Autodesk Fusion 360 part; units mm, degrees
note: some values were not read from the file. Set by a fixed rule: which sketch regions a step uses.
(part 7 of 14)
  spline S34 degree 5 poles (16.842, -9.555) (16.8421, -9.5551) (16.8422, -9.5551) (16.8424, -9.5553) (16.8428, -9.5555) (16.8433, -9.5558) (16.8439, -9.5561) (16.8446, -9.5565) (16.8454, -9.5569) (16.8462, -9.5573) (16.8472, -9.5578) (16.8482, -9.5584) (16.8493, -9.5589) (16.8504, -9.5596) (16.8517, -9.5602) (16.853, -9.5609) (16.8544, -9.5616) (16.8558, -9.5624) (16.8574, -9.5631) (16.859, -9.564) (16.8606, -9.5648) (16.8624, -9.5657) (16.8642, -9.5666) (16.8661, -9.5676) (16.8681, -9.5685) (16.8701, -9.5695) (16.8722, -9.5706) (16.8744, -9.5716) (16.8766, -9.5727) (16.8789, -9.5739) (16.8813, -9.575) (16.8837, -9.5762) (16.8863, -9.5774) (16.8888, -9.5786) (16.8915, -9.5798) (16.8942, -9.5811) (16.897, -9.5824) (16.8998, -9.5837) (16.9027, -9.5851) (16.9057, -9.5864) (16.9087, -9.5878) (16.9118, -9.5892) (16.9149, -9.5906) (16.9182, -9.5921) (16.9214, -9.5936) (16.9248, -9.5951) (16.9282, -9.5966) (16.9316, -9.5981) (16.9352, -9.5996) (16.9387, -9.6012) (16.9424, -9.6028) (16.9461, -9.6044) (16.9499, -9.606) (16.9537, -9.6076) (16.9576, -9.6093) (16.9615, -9.6109) (16.9655, -9.6126) (16.9695, -9.6143) (16.9737, -9.616) (16.9778, -9.6177) (16.982, -9.6195) (16.9863, -9.6212) (16.9907, -9.623) (16.9951, -9.6248) (16.9995, -9.6266) (17.004, -9.6284) (17.0086, -9.6302) (17.0132, -9.632) (17.0178, -9.6339) (17.0226, -9.6357) (17.0273, -9.6376) (17.0322, -9.6395) (17.0371, -9.6413) (17.042, -9.6432) (17.047, -9.6451) (17.052, -9.6471) (17.0571, -9.649) (17.0623, -9.6509) (17.0675, -9.6528) (17.0727, -9.6548) (17.078, -9.6568) (17.0834, -9.6587) (17.0888, -9.6607) (17.0942, -9.6627) (17.0997, -9.6647) (17.1053, -9.6667) (17.1109, -9.6687) (17.1166, -9.6707) (17.1223, -9.6727) (17.128, -9.6747) (17.1338, -9.6767) (17.1397, -9.6788) (17.1456, -9.6808) (17.1515, -9.6828) (17.1575, -9.6849) (17.1636, -9.6869) (17.1697, -9.689) (17.1758, -9.6911) (17.182, -9.6931) (17.1882, -9.6952) (17.1945, -9.6973) (17.2009, -9.6993) (17.2072, -9.7014) (17.2137, -9.7035) (17.2201, -9.7056) (17.2267, -9.7077) (17.2332, -9.7098) (17.2398, -9.7119) (17.2465, -9.714) (17.2532, -9.7161) (17.2599, -9.7181) (17.2667, -9.7202) (17.2736, -9.7223) (17.2805, -9.7244) (17.2874, -9.7265) (17.2944, -9.7287) (17.3014, -9.7308) (17.3084, -9.7329) (17.3155, -9.735) (17.3227, -9.7371) (17.3299, -9.7392) (17.3371, -9.7413) (17.3444, -9.7434) (17.3517, -9.7455) (17.3591, -9.7476) (17.3665, -9.7497) (17.3739, -9.7518) (17.3814, -9.7539) (17.389, -9.756) (17.3966, -9.7581) (17.4042, -9.7602) (17.4118, -9.7622) (17.4195, -9.7643) (17.4273, -9.7664) (17.4351, -9.7685) (17.4429, -9.7706) (17.4508, -9.7727) (17.4587, -9.7747) (17.4666, -9.7768) (17.4746, -9.7789) (17.4827, -9.7809) (17.4907, -9.783) (17.4988, -9.785) (17.507, -9.7871) (17.5152, -9.7892) (17.5234, -9.7912) (17.5317, -9.7932) (17.54, -9.7953) (17.5484, -9.7973) (17.5568, -9.7993) (17.5652, -9.8014) (17.5737, -9.8034) (17.5822, -9.8054) (17.5907, -9.8074) (17.5993, -9.8094) (17.6079, -9.8114) (17.6166, -9.8134) (17.6253, -9.8154) (17.634, -9.8174) (17.6428, -9.8193) (17.6516, -9.8213) (17.6605, -9.8233) (17.6694, -9.8252) (17.6783, -9.8272) (17.6873, -9.8291) (17.6963, -9.831) (17.7053, -9.833) (17.7144, -9.8349) (17.7235, -9.8368) (17.7326, -9.8387) (17.7418, -9.8406) (17.751, -9.8425) (17.7603, -9.8444) (17.7696, -9.8463) (17.7789, -9.8481) (17.7883, -9.85) (17.7977, -9.8519) (17.8071, -9.8537) (17.8166, -9.8555) (17.8261, -9.8574) (17.8357, -9.8592) (17.8453, -9.861) (17.8549, -9.8628) (17.8645, -9.8646) (17.8742, -9.8664) (17.8839, -9.8682) (17.8937, -9.8699) (17.9035, -9.8717) (17.9133, -9.8735) (17.9232, -9.8752) (17.9331, -9.8769) (17.943, -9.8787) (17.9529, -9.8804) (17.9629, -9.8821) (17.973, -9.8838) (17.983, -9.8855) (17.9931, -9.8871) (18.0033, -9.8888) (18.0134, -9.8904) (18.0236, -9.8921) (18.0339, -9.8937) (18.0441, -9.8953) (18.0544, -9.897) (18.0647, -9.8986) (18.0751, -9.9002) (18.0855, -9.9017) (18.0959, -9.9033) (18.1064, -9.9049) (18.1169, -9.9064) (18.1274, -9.9079) (18.138, -9.9095) (18.1486, -9.911) (18.1592, -9.9125) (18.1698, -9.914) (18.1805, -9.9155) (18.1912, -9.9169) (18.202, -9.9184) (18.2128, -9.9198) (18.2236, -9.9213) (18.2344, -9.9227) (18.2453, -9.9241) (18.2562, -9.9255) (18.2671, -9.9269) (18.2781, -9.9282) (18.2891, -9.9296) (18.3001, -9.9309) (18.3112, -9.9323) (18.3223, -9.9336) (18.3334, -9.9349) (18.3445, -9.9362) (18.3557, -9.9375) (18.3669, -9.9387) (18.3782, -9.94) (18.3894, -9.9412) (18.4007, -9.9425) (18.4121, -9.9437) (18.4234, -9.9449) (18.4348, -9.9461) (18.4462, -9.9473) (18.4577, -9.9484) (18.4691, -9.9496) (18.4783, -9.9505) (18.4853, -9.9512) (18.4899, -9.9516) (18.4922, -9.9518) knots 0 0 0 0 0 0 0.00416667 0.00833333 0.0125 0.01666667 0.02083333 0.025 0.02916667 0.03333333 0.0375 0.04166667 0.04583333 0.05 0.05416667 0.05833333 0.0625 0.06666667 0.07083333 0.075 0.07916667 0.08333333 0.0875 0.09166667 0.09583333 0.1 0.10416667 0.10833333 0.1125 0.11666667 0.12083333 0.125 0.12916667 0.13333333 0.1375 0.14166667 0.14583333 0.15 0.15416667 0.15833333 0.1625 0.16666667 0.17083333 0.175 0.17916667 0.18333333 0.1875 0.19166667 0.19583333 0.2 0.20416667 0.20833333 0.2125 0.21666667 0.22083333 0.225 0.22916667 0.23333333 0.2375 0.24166667 0.24583333 0.25 0.25416667 0.25833333 0.2625 0.26666667 0.27083333 0.275 0.27916667 0.28333333 0.2875 0.29166667 0.29583333 0.3 0.30416667 0.30833333 0.3125 0.31666667 0.32083333 0.325 0.32916667 0.33333333 0.3375 0.34166667 0.34583333 0.35 0.35416667 0.35833333 0.3625 0.36666667 0.37083333 0.375 0.37916667 0.38333333 0.3875 0.39166667 0.39583333 0.4 0.40416667 0.40833333 0.4125 0.41666667 0.42083333 0.425 0.42916667 0.43333333 0.4375 0.44166667 0.44583333 0.45 0.45416667 0.45833333 0.4625 0.46666667 0.47083333 0.475 0.47916667 0.48333333 0.4875 0.49166667 0.49583333 0.5 0.50416667 0.50833333 0.5125 0.51666667 0.52083333 0.525 0.52916667 0.53333333 0.5375 0.54166667 0.54583333 0.55 0.55416667 0.55833333 0.5625 0.56666667 0.57083333 0.575 0.57916667 0.58333333 0.5875 0.59166667 0.59583333 0.6 0.60416667 0.60833333 0.6125 0.61666667 0.62083333 0.625 0.62916667 0.63333333 0.6375 0.64166667 0.64583333 0.65 0.65416667 0.65833333 0.6625 0.66666667 0.67083333 0.675 0.67916667 0.68333333 0.6875 0.69166667 0.69583333 0.7 0.70416667 0.70833333 0.7125 0.71666667 0.72083333 0.725 0.72916667 0.73333333 0.7375 0.74166667 0.74583333 0.75 0.75416667 0.75833333 0.7625 0.76666667 0.77083333 0.775 0.77916667 0.78333333 0.7875 0.79166667 0.79583333 0.8 0.80416667 0.80833333 0.8125 0.81666667 0.82083333 0.825 0.82916667 0.83333333 0.8375 0.84166667 0.84583333 0.85 0.85416667 0.85833333 0.8625 0.86666667 0.87083333 0.875 0.87916667 0.88333333 0.8875 0.89166667 0.89583333 0.9 0.90416667 0.90833333 0.9125 0.91666667 0.92083333 0.925 0.92916667 0.93333333 0.9375 0.94166667 0.94583333 0.95 0.95416667 0.95833333 0.9625 0.96666667 0.97083333 0.975 0.97916667 0.98333333 0.9875 0.99166667 0.99583333 1 1 1 1 1 1
  arc A35 (18.4922, -9.9518) -> (18.9206, -9.111) centre (0, 0) ccw
  spline S35 degree 5 poles (18.9206, -9.111) (18.9191, -9.1092) (18.916, -9.1058) (18.9114, -9.1006) (18.9053, -9.0936) (18.8976, -9.085) (18.8899, -9.0765) (18.8823, -9.0679) (18.8746, -9.0594) (18.8669, -9.0509) (18.8593, -9.0425) (18.8517, -9.034) (18.844, -9.0257) (18.8364, -9.0173) (18.8288, -9.009) (18.8212, -9.0007) (18.8136, -8.9924) (18.806, -8.9842) (18.7984, -8.976) (18.7908, -8.9678) (18.7833, -8.9597) (18.7757, -8.9516) (18.7681, -8.9436) (18.7606, -8.9355) (18.7531, -8.9275) (18.7455, -8.9195) (18.738, -8.9116) (18.7305, -8.9037) (18.723, -8.8958) (18.7155, -8.888) (18.708, -8.8802) (18.7005, -8.8724) (18.6931, -8.8647) (18.6856, -8.857) (18.6782, -8.8493) (18.6707, -8.8416) (18.6633, -8.834) (18.6559, -8.8264) (18.6485, -8.8189) (18.6411, -8.8114) (18.6337, -8.8039) (18.6263, -8.7965) (18.6189, -8.789) (18.6116, -8.7817) (18.6042, -8.7743) (18.5969, -8.767) (18.5896, -8.7597) (18.5823, -8.7525) (18.575, -8.7452) (18.5677, -8.7381) (18.5604, -8.7309) (18.5531, -8.7238) (18.5459, -8.7167) (18.5386, -8.7096) (18.5314, -8.7026) (18.5242, -8.6956) (18.517, -8.6887) (18.5098, -8.6818) (18.5026, -8.6749) (18.4954, -8.668) (18.4883, -8.6612) (18.4811, -8.6544) (18.474, -8.6477) (18.4669, -8.641) (18.4598, -8.6343) (18.4527, -8.6276) (18.4456, -8.621) (18.4386, -8.6144) (18.4315, -8.6079) (18.4245, -8.6013) (18.4175, -8.5949) (18.4105, -8.5884) (18.4035, -8.582) (18.3966, -8.5756) (18.3896, -8.5693) (18.3827, -8.5629) (18.3757, -8.5567) (18.3688, -8.5504) (18.3619, -8.5442) (18.3551, -8.538) (18.3482, -8.5319) (18.3414, -8.5258) (18.3346, -8.5197) (18.3277, -8.5137) (18.321, -8.5076) (18.3142, -8.5017) (18.3074, -8.4957) (18.3007, -8.4898) (18.294, -8.4839) (18.2873, -8.4781) (18.2806, -8.4723) (18.2739, -8.4665) (18.2673, -8.4608) (18.2606, -8.4551) (18.254, -8.4494) (18.2474, -8.4438) (18.2409, -8.4382) (18.2343, -8.4326) (18.2278, -8.4271) (18.2213, -8.4216) (18.2148, -8.4162) (18.2083, -8.4107) (18.2018, -8.4054) (18.1954, -8.4) (18.189, -8.3947) (18.1826, -8.3894) (18.1762, -8.3841) (18.1699, -8.3789) (18.1635, -8.3737) (18.1572, -8.3686) (18.151, -8.3635) (18.1447, -8.3584) (18.1385, -8.3534) (18.1322, -8.3484) (18.126, -8.3434) (18.1199, -8.3385) (18.1137, -8.3336) (18.1076, -8.3287) (18.1015, -8.3239) (18.0954, -8.3191) (18.0894, -8.3143) (18.0833, -8.3096) (18.0773, -8.3049) (18.0714, -8.3003) (18.0654, -8.2956) (18.0595, -8.291) (18.0536, -8.2865) (18.0477, -8.282) (18.0418, -8.2775) (18.036, -8.2731) (18.0302, -8.2687) (18.0244, -8.2643) (18.0187, -8.26) (18.013, -8.2557) (18.0073, -8.2514) (18.0016, -8.2472) (17.996, -8.243) (17.9904, -8.2388) (17.9848, -8.2347) (17.9793, -8.2306) (17.9737, -8.2266) (17.9682, -8.2226) (17.9628, -8.2186) (17.9573, -8.2147) (17.9519, -8.2108) (17.9466, -8.2069) (17.9412, -8.2031) (17.9359, -8.1993) (17.9306, -8.1955) (17.9254, -8.1918) (17.9202, -8.1881) (17.915, -8.1844) (17.9098, -8.1808) (17.9047, -8.1772) (17.8996, -8.1737) (17.8946, -8.1702) (17.8896, -8.1667) (17.8846, -8.1633) (17.8796, -8.1599) (17.8747, -8.1565) (17.8698, -8.1532) (17.865, -8.1499) (17.8602, -8.1467) (17.8554, -8.1435) (17.8507, -8.1403) (17.846, -8.1372) (17.8413, -8.1341) (17.8367, -8.131) (17.8321, -8.128) (17.8276, -8.125) (17.823, -8.122) (17.8186, -8.1191) (17.8141, -8.1162) (17.8097, -8.1134) (17.8054, -8.1106) (17.8011, -8.1078) (17.7968, -8.1051) (17.7926, -8.1024) (17.7884, -8.0997) (17.7842, -8.0971) (17.7801, -8.0945) (17.7761, -8.092) (17.772, -8.0895) (17.7681, -8.087) (17.7641, -8.0846) (17.7602, -8.0822) (17.7564, -8.0798) (17.7526, -8.0775) (17.7488, -8.0752) (17.7451, -8.073) (17.7415, -8.0708) (17.7378, -8.0686) (17.7343, -8.0665) (17.7308, -8.0644) (17.7273, -8.0623) (17.7239, -8.0603) (17.7205, -8.0583) (17.7172, -8.0564) (17.7139, -8.0545) (17.7107, -8.0526) (17.7075, -8.0508) (17.7044, -8.049) (17.7013, -8.0472) (17.6983, -8.0455) (17.6954, -8.0438) (17.6925, -8.0422) (17.6896, -8.0406) (17.6868, -8.0391) (17.6841, -8.0375) (17.6814, -8.0361) (17.6788, -8.0346) (17.6762, -8.0332) (17.6737, -8.0318) (17.6713, -8.0305) (17.6689, -8.0292) (17.6666, -8.028) (17.6643, -8.0268) (17.6621, -8.0256) (17.66, -8.0245) (17.6579, -8.0234) (17.6559, -8.0223) (17.654, -8.0213) (17.6521, -8.0203) (17.6503, -8.0194) (17.6485, -8.0185) (17.6469, -8.0176) (17.6452, -8.0168) (17.6437, -8.016) (17.6422, -8.0153) (17.6408, -8.0146) (17.6395, -8.0139) (17.6383, -8.0133) (17.6371, -8.0127) (17.636, -8.0122) (17.635, -8.0117) (17.634, -8.0112) (17.6332, -8.0108) (17.6324, -8.0104) (17.6317, -8.0101) (17.631, -8.0098) (17.6305, -8.0095) (17.6301, -8.0094) (17.6299, -8.0093) (17.6297, -8.0092) (17.6297, -8.0092) knots -1 -1 -1 -1 -1 -1 -0.99583333 -0.99166667 -0.9875 -0.98333333 -0.97916667 -0.975 -0.97083333 -0.96666667 -0.9625 -0.95833333 -0.95416667 -0.95 -0.94583333 -0.94166667 -0.9375 -0.93333333 -0.92916667 -0.925 -0.92083333 -0.91666667 -0.9125 -0.90833333 -0.90416667 -0.9 -0.89583333 -0.89166667 -0.8875 -0.88333333 -0.87916667 -0.875 -0.87083333 -0.86666667 -0.8625 -0.85833333 -0.85416667 -0.85 -0.84583333 -0.84166667 -0.8375 -0.83333333 -0.82916667 -0.825 -0.82083333 -0.81666667 -0.8125 -0.80833333 -0.80416667 -0.8 -0.79583333 -0.79166667 -0.7875 -0.78333333 -0.77916667 -0.775 -0.77083333 -0.76666667 -0.7625 -0.75833333 -0.75416667 -0.75 -0.74583333 -0.74166667 -0.7375 -0.73333333 -0.72916667 -0.725 -0.72083333 -0.71666667 -0.7125 -0.70833333 -0.70416667 -0.7 -0.69583333 -0.69166667 -0.6875 -0.68333333 -0.67916667 -0.675 -0.67083333 -0.66666667 -0.6625 -0.65833333 -0.65416667 -0.65 -0.64583333 -0.64166667 -0.6375 -0.63333333 -0.62916667 -0.625 -0.62083333 -0.61666667 -0.6125 -0.60833333 -0.60416667 -0.6 -0.59583333 -0.59166667 -0.5875 -0.58333333 -0.57916667 -0.575 -0.57083333 -0.56666667 -0.5625 -0.55833333 -0.55416667 -0.55 -0.54583333 -0.54166667 -0.5375 -0.53333333 -0.52916667 -0.525 -0.52083333 -0.51666667 -0.5125 -0.50833333 -0.50416667 -0.5 -0.49583333 -0.49166667 -0.4875 -0.48333333 -0.47916667 -0.475 -0.47083333 -0.46666667 -0.4625 -0.45833333 -0.45416667 -0.45 -0.44583333 -0.44166667 -0.4375 -0.43333333 -0.42916667 -0.425 -0.42083333 -0.41666667 -0.4125 -0.40833333 -0.40416667 -0.4 -0.39583333 -0.39166667 -0.3875 -0.38333333 -0.37916667 -0.375 -0.37083333 -0.36666667 -0.3625 -0.35833333 -0.35416667 -0.35 -0.34583333 -0.34166667 -0.3375 -0.33333333 -0.32916667 -0.325 -0.32083333 -0.31666667 -0.3125 -0.30833333 -0.30416667 -0.3 -0.29583333 -0.29166667 -0.2875 -0.28333333 -0.27916667 -0.275 -0.27083333 -0.26666667 -0.2625 -0.25833333 -0.25416667 -0.25 -0.24583333 -0.24166667 -0.2375 -0.23333333 -0.22916667 -0.225 -0.22083333 -0.21666667 -0.2125 -0.20833333 -0.20416667 -0.2 -0.19583333 -0.19166667 -0.1875 -0.18333333 -0.17916667 -0.175 -0.17083333 -0.16666667 -0.1625 -0.15833333 -0.15416667 -0.15 -0.14583333 -0.14166667 -0.1375 -0.13333333 -0.12916667 -0.125 -0.12083333 -0.11666667 -0.1125 -0.10833333 -0.10416667 -0.1 -0.09583333 -0.09166667 -0.0875 -0.08333333 -0.07916667 -0.075 -0.07083333 -0.06666667 -0.0625 -0.05833333 -0.05416667 -0.05 -0.04583333 -0.04166667 -0.0375 -0.03333333 -0.02916667 -0.025 -0.02083333 -0.01666667 -0.0125 -0.00833333 -0.00416667 0 0 0 0 0 0
  line L70 (17.6297, -8.0092) -> (17.629, -8.0089)
  line L71 (17.629, -8.0089) -> (17.0709, -7.7553)
  arc A36 (17.0709, -7.7553) -> (17.5548, -6.5871) centre (0, 0) ccw
  line L72 (17.5548, -6.5871) -> (18.1287, -6.8025)
  line L73 (18.1287, -6.8025) -> (18.1294, -6.8027)
  spline S36 degree 5 poles (18.1294, -6.8027) (18.1295, -6.8027) (18.1296, -6.8028) (18.1298, -6.8029) (18.1302, -6.803) (18.1308, -6.8032) (18.1315, -6.8035) (18.1322, -6.8037) (18.133, -6.804) (18.1339, -6.8043) (18.1349, -6.8047) (18.136, -6.8051) (18.1372, -6.8055) (18.1384, -6.8059) (18.1397, -6.8063) (18.1411, -6.8068) (18.1426, -6.8073) (18.1442, -6.8078) (18.1458, -6.8083) (18.1475, -6.8089) (18.1493, -6.8095) (18.1512, -6.8101) (18.1531, -6.8107) (18.1552, -6.8113) (18.1572, -6.812) (18.1594, -6.8127) (18.1617, -6.8134) (18.164, -6.8141) (18.1663, -6.8148) (18.1688, -6.8155) (18.1713, -6.8163) (18.1739, -6.8171) (18.1766, -6.8179) (18.1793, -6.8187) (18.1821, -6.8195) (18.185, -6.8203) (18.1879, -6.8212) (18.191, -6.822) (18.194, -6.8229) (18.1972, -6.8238) (18.2004, -6.8247) (18.2037, -6.8256) (18.207, -6.8265) (18.2104, -6.8274) (18.2139, -6.8284) (18.2174, -6.8293) (18.221, -6.8303) (18.2247, -6.8312) (18.2284, -6.8322) (18.2322, -6.8332) (18.236, -6.8342) (18.2399, -6.8352) (18.2439, -6.8362) (18.2479, -6.8372) (18.252, -6.8382) (18.2561, -6.8392) (18.2604, -6.8403) (18.2646, -6.8413) (18.269, -6.8424) (18.2733, -6.8434) (18.2778, -6.8445) (18.2823, -6.8455) (18.2868, -6.8466) (18.2915, -6.8477) (18.2961, -6.8487) (18.3009, -6.8498) (18.3057, -6.8509) (18.3105, -6.852) (18.3154, -6.8531) (18.3203, -6.8542) (18.3254, -6.8553) (18.3304, -6.8564) (18.3355, -6.8575) (18.3407, -6.8586) (18.3459, -6.8597) (18.3512, -6.8608) (18.3565, -6.8619) (18.3619, -6.863) (18.3674, -6.8641) (18.3729, -6.8652) (18.3784, -6.8663) (18.384, -6.8674) (18.3896, -6.8685) (18.3953, -6.8696) (18.4011, -6.8707) (18.4069, -6.8718) (18.4127, -6.8729) (18.4186, -6.874) (18.4246, -6.8751) (18.4306, -6.8762) (18.4366, -6.8773) (18.4427, -6.8784) (18.4489, -6.8795) (18.4551, -6.8805) (18.4613, -6.8816) (18.4676, -6.8827) (18.474, -6.8838) (18.4804, -6.8849) (18.4868, -6.8859) (18.4933, -6.887) (18.4998, -6.8881) (18.5064, -6.8891) (18.513, -6.8902) (18.5197, -6.8912) (18.5264, -6.8923) (18.5332, -6.8933) (18.54, -6.8944) (18.5469, -6.8954) (18.5538, -6.8964) (18.5607, -6.8974) (18.5677, -6.8985) (18.5747, -6.8995) (18.5818, -6.9005) (18.5889, -6.9015) (18.5961, -6.9025) (18.6033, -6.9034) (18.6106, -6.9044) (18.6179, -6.9054) (18.6252, -6.9064) (18.6326, -6.9073) (18.6401, -6.9083) (18.6475, -6.9092) (18.6551, -6.9102) (18.6626, -6.9111) (18.6702, -6.912) (18.6779, -6.9129) (18.6856, -6.9138) (18.6933, -6.9147) (18.7011, -6.9156) (18.7089, -6.9165) (18.7167, -6.9174) (18.7246, -6.9182) (18.7326, -6.9191) (18.7405, -6.9199) (18.7485, -6.9208) (18.7566, -6.9216) (18.7647, -6.9224) (18.7728, -6.9232) (18.781, -6.924) (18.7892, -6.9248) (18.7975, -6.9256) (18.8058, -6.9264) (18.8141, -6.9272) (18.8225, -6.9279) (18.8309, -6.9287) (18.8394, -6.9294) (18.8479, -6.9301) (18.8564, -6.9308) (18.8649, -6.9315) (18.8736, -6.9322) (18.8822, -6.9329) (18.8909, -6.9336) (18.8996, -6.9342) (18.9084, -6.9349) (18.9171, -6.9355) (18.926, -6.9361) (18.9348, -6.9367) (18.9438, -6.9373) (18.9527, -6.9379) (18.9617, -6.9385) (18.9707, -6.9391) (18.9797, -6.9396) (18.9888, -6.9402) (18.9979, -6.9407) (19.0071, -6.9412) (19.0163, -6.9417) (19.0255, -6.9422) (19.0348, -6.9427) (19.0441, -6.9431) (19.0534, -6.9436) (19.0628, -6.944) (19.0722, -6.9445) (19.0816, -6.9449) (19.0911, -6.9453) (19.1006, -6.9457) (19.1102, -6.946) (19.1198, -6.9464) (19.1294, -6.9467) (19.139, -6.9471) (19.1487, -6.9474) (19.1584, -6.9477) (19.1681, -6.948) (19.1779, -6.9483) (19.1877, -6.9485) (19.1976, -6.9488) (19.2075, -6.949) (19.2174, -6.9492) (19.2273, -6.9495) (19.2373, -6.9496) (19.2473, -6.9498) (19.2574, -6.95) (19.2674, -6.9501) (19.2775, -6.9503) (19.2877, -6.9504) (19.2979, -6.9505) (19.3081, -6.9506) (19.3183, -6.9507) (19.3286, -6.9507) (19.3389, -6.9508) (19.3492, -6.9508) (19.3595, -6.9508) (19.3699, -6.9508) (19.3804, -6.9508) (19.3908, -6.9507) (19.4013, -6.9507) (19.4118, -6.9506) (19.4224, -6.9505) (19.4329, -6.9505) (19.4435, -6.9503) (19.4542, -6.9502) (19.4648, -6.9501) (19.4755, -6.9499) (19.4863, -6.9497) (19.497, -6.9495) (19.5078, -6.9493) (19.5186, -6.9491) (19.5295, -6.9488) (19.5403, -6.9486) (19.5512, -6.9483) (19.5622, -6.948) (19.5731, -6.9477) (19.5841, -6.9474) (19.5951, -6.947) (19.6062, -6.9467) (19.6172, -6.9463) (19.6283, -6.9459) (19.6395, -6.9455) (19.6506, -6.9451) (19.6618, -6.9446) (19.673, -6.9441) (19.6843, -6.9437) (19.6956, -6.9432) (19.7068, -6.9426) (19.7182, -6.9421) (19.7295, -6.9416) (19.7409, -6.941) (19.7523, -6.9404) (19.7637, -6.9398) (19.7752, -6.9392) (19.7867, -6.9385) (19.7982, -6.9379) (19.8074, -6.9373) (19.8144, -6.9369) (19.819, -6.9366) (19.8213, -6.9365) knots 0 0 0 0 0 0 0.00416667 0.00833333 0.0125 0.01666667 0.02083333 0.025 0.02916667 0.03333333 0.0375 0.04166667 0.04583333 0.05 0.05416667 0.05833333 0.0625 0.06666667 0.07083333 0.075 0.07916667 0.08333333 0.0875 0.09166667 0.09583333 0.1 0.10416667 0.10833333 0.1125 0.11666667 0.12083333 0.125 0.12916667 0.13333333 0.1375 0.14166667 0.14583333 0.15 0.15416667 0.15833333 0.1625 0.16666667 0.17083333 0.175 0.17916667 0.18333333 0.1875 0.19166667 0.19583333 0.2 0.20416667 0.20833333 0.2125 0.21666667 0.22083333 0.225 0.22916667 0.23333333 0.2375 0.24166667 0.24583333 0.25 0.25416667 0.25833333 0.2625 0.26666667 0.27083333 0.275 0.27916667 0.28333333 0.2875 0.29166667 0.29583333 0.3 0.30416667 0.30833333 0.3125 0.31666667 0.32083333 0.325 0.32916667 0.33333333 0.3375 0.34166667 0.34583333 0.35 0.35416667 0.35833333 0.3625 0.36666667 0.37083333 0.375 0.37916667 0.38333333 0.3875 0.39166667 0.39583333 0.4 0.40416667 0.40833333 0.4125 0.41666667 0.42083333 0.425 0.42916667 0.43333333 0.4375 0.44166667 0.44583333 0.45 0.45416667 0.45833333 0.4625 0.46666667 0.47083333 0.475 0.47916667 0.48333333 0.4875 0.49166667 0.49583333 0.5 0.50416667 0.50833333 0.5125 0.51666667 0.52083333 0.525 0.52916667 0.53333333 0.5375 0.54166667 0.54583333 0.55 0.55416667 0.55833333 0.5625 0.56666667 0.57083333 0.575 0.57916667 0.58333333 0.5875 0.59166667 0.59583333 0.6 0.60416667 0.60833333 0.6125 0.61666667 0.62083333 0.625 0.62916667 0.63333333 0.6375 0.64166667 0.64583333 0.65 0.65416667 0.65833333 0.6625 0.66666667 0.67083333 0.675 0.67916667 0.68333333 0.6875 0.69166667 0.69583333 0.7 0.70416667 0.70833333 0.7125 0.71666667 0.72083333 0.725 0.72916667 0.73333333 0.7375 0.74166667 0.74583333 0.75 0.75416667 0.75833333 0.7625 0.76666667 0.77083333 0.775 0.77916667 0.78333333 0.7875 0.79166667 0.79583333 0.8 0.80416667 0.80833333 0.8125 0.81666667 0.82083333 0.825 0.82916667 0.83333333 0.8375 0.84166667 0.84583333 0.85 0.85416667 0.85833333 0.8625 0.86666667 0.87083333 0.875 0.87916667 0.88333333 0.8875 0.89166667 0.89583333 0.9 0.90416667 0.90833333 0.9125 0.91666667 0.92083333 0.925 0.92916667 0.93333333 0.9375 0.94166667 0.94583333 0.95 0.95416667 0.95833333 0.9625 0.96666667 0.97083333 0.975 0.97916667 0.98333333 0.9875 0.99166667 0.99583333 1 1 1 1 1 1
  arc A37 (19.8213, -6.9365) -> (20.113, -6.039) centre (0, 0) ccw
  spline S37 degree 5 poles (20.113, -6.039) (20.1112, -6.0375) (20.1076, -6.0345) (20.1022, -6.0301) (20.0951, -6.0242) (20.0861, -6.0169) (20.0772, -6.0097) (20.0683, -6.0024) (20.0594, -5.9952) (20.0505, -5.988) (20.0417, -5.9809) (20.0328, -5.9738) (20.024, -5.9667) (20.0151, -5.9596) (20.0063, -5.9526) (19.9975, -5.9456) (19.9887, -5.9386) (19.9799, -5.9317) (19.9711, -5.9248) (19.9624, -5.9179) (19.9536, -5.9111) (19.9449, -5.9042) (19.9362, -5.8975) (19.9274, -5.8907) (19.9187, -5.884) (19.9101, -5.8773) (19.9014, -5.8706) (19.8927, -5.864) (19.8841, -5.8574) (19.8755, -5.8508) (19.8668, -5.8443) (19.8582, -5.8378) (19.8497, -5.8313) (19.8411, -5.8248) (19.8325, -5.8184) (19.824, -5.812) (19.8155, -5.8057) (19.8069, -5.7994) (19.7984, -5.7931) (19.79, -5.7868) (19.7815, -5.7806) (19.773, -5.7744) (19.7646, -5.7682) (19.7562, -5.7621) (19.7478, -5.7559) (19.7394, -5.7499) (19.731, -5.7438) (19.7227, -5.7378) (19.7143, -5.7318) (19.706, -5.7259) (19.6977, -5.7199) (19.6894, -5.714) (19.6811, -5.7082) (19.6729, -5.7023) (19.6646, -5.6965) (19.6564, -5.6908) (19.6482, -5.685) (19.64, -5.6793) (19.6319, -5.6736) (19.6237, -5.668) (19.6156, -5.6624) (19.6075, -5.6568) (19.5994, -5.6512) (19.5913, -5.6457) (19.5832, -5.6402) (19.5752, -5.6348) (19.5672, -5.6293) (19.5592, -5.6239) (19.5512, -5.6186) (19.5432, -5.6132) (19.5353, -5.6079) (19.5274, -5.6026) (19.5195, -5.5974) (19.5116, -5.5922) (19.5037, -5.587) (19.4959, -5.5818) (19.4881, -5.5767) (19.4803, -5.5716) (19.4725, -5.5666) (19.4647, -5.5615) (19.457, -5.5565) (19.4493, -5.5516) (19.4416, -5.5466) (19.4339, -5.5417) (19.4263, -5.5369) (19.4187, -5.532) (19.4111, -5.5272) (19.4035, -5.5224) (19.3959, -5.5177) (19.3884, -5.513) (19.3809, -5.5083) (19.3734, -5.5036) (19.3659, -5.499) (19.3585, -5.4944) (19.3511, -5.4899) (19.3437, -5.4853) (19.3363, -5.4808) (19.329, -5.4764) (19.3216, -5.4719) (19.3144, -5.4675) (19.3071, -5.4631) (19.2998, -5.4588) (19.2926, -5.4545) (19.2854, -5.4502) (19.2783, -5.4459) (19.2711, -5.4417) (19.264, -5.4375) (19.2569, -5.4334) (19.2499, -5.4293) (19.2428, -5.4252) (19.2358, -5.4211) (19.2288, -5.4171) (19.2219, -5.4131) (19.215, -5.4091) (19.2081, -5.4051) (19.2012, -5.4012) (19.1944, -5.3974) (19.1876, -5.3935) (19.1808, -5.3897) (19.174, -5.3859) (19.1673, -5.3822) (19.1606, -5.3784) (19.1539, -5.3747) (19.1473, -5.3711) (19.1407, -5.3674) (19.1341, -5.3638) (19.1276, -5.3603) (19.1211, -5.3567) (19.1146, -5.3532) (19.1082, -5.3498) (19.1017, -5.3463) (19.0954, -5.3429) (19.089, -5.3395) (19.0827, -5.3362) (19.0764, -5.3329) (19.0701, -5.3296) (19.0639, -5.3263) (19.0577, -5.3231) (19.0516, -5.3199) (19.0455, -5.3167) (19.0394, -5.3136) (19.0333, -5.3105) (19.0273, -5.3074) (19.0213, -5.3044) (19.0154, -5.3014) (19.0095, -5.2984) (19.0036, -5.2954) (18.9978, -5.2925) (18.9919, -5.2896) (18.9862, -5.2868) (18.9805, -5.2839) (18.9748, -5.2812) (18.9691, -5.2784) (18.9635, -5.2757) (18.9579, -5.273) (18.9524, -5.2703) (18.9469, -5.2676) (18.9414, -5.265) (18.936, -5.2625) (18.9306, -5.2599) (18.9253, -5.2574) (18.92, -5.2549) (18.9147, -5.2524) (18.9095, -5.25) (18.9043, -5.2476) (18.8992, -5.2453) (18.8941, -5.2429) (18.8891, -5.2406) (18.8841, -5.2383) (18.8791, -5.2361) (18.8742, -5.2339) (18.8693, -5.2317) (18.8645, -5.2296) (18.8597, -5.2274) (18.8549, -5.2253) (18.8503, -5.2233) (18.8456, -5.2213) (18.841, -5.2193) (18.8364, -5.2173) (18.8319, -5.2154) (18.8275, -5.2134) (18.8231, -5.2116) (18.8187, -5.2097) (18.8144, -5.2079) (18.8101, -5.2061) (18.8059, -5.2044) (18.8017, -5.2026) (18.7976, -5.2009) (18.7936, -5.1993) (18.7895, -5.1976) (18.7856, -5.196) (18.7817, -5.1944) (18.7778, -5.1929) (18.774, -5.1914) (18.7703, -5.1899) (18.7666, -5.1884) (18.7629, -5.187) (18.7593, -5.1856) (18.7558, -5.1842) (18.7523, -5.1829) (18.7489, -5.1816) (18.7456, -5.1803) (18.7423, -5.1791) (18.739, -5.1778) (18.7359, -5.1766) (18.7327, -5.1755) (18.7297, -5.1744) (18.7267, -5.1732) (18.7237, -5.1722) (18.7209, -5.1711) (18.718, -5.1701) (18.7153, -5.1691) (18.7126, -5.1682) (18.71, -5.1672) (18.7074, -5.1663) (18.7049, -5.1655) (18.7025, -5.1646) (18.7002, -5.1638) (18.6979, -5.163) (18.6957, -5.1623) (18.6935, -5.1615) (18.6914, -5.1608) (18.6894, -5.1602) (18.6875, -5.1595) (18.6856, -5.1589) (18.6838, -5.1583) (18.6821, -5.1578) (18.6805, -5.1573) (18.6789, -5.1568) (18.6774, -5.1563) (18.676, -5.1558) (18.6747, -5.1554) (18.6734, -5.155) (18.6723, -5.1547) (18.6712, -5.1543) (18.6702, -5.154) (18.6692, -5.1538) (18.6684, -5.1535) (18.6676, -5.1533) (18.667, -5.1531) (18.6664, -5.1529) (18.666, -5.1528) (18.6657, -5.1527) (18.6656, -5.1527) (18.6655, -5.1527) knots -1 -1 -1 -1 -1 -1 -0.99583333 -0.99166667 -0.9875 -0.98333333 -0.97916667 -0.975 -0.97083333 -0.96666667 -0.9625 -0.95833333 -0.95416667 -0.95 -0.94583333 -0.94166667 -0.9375 -0.93333333 -0.92916667 -0.925 -0.92083333 -0.91666667 -0.9125 -0.90833333 -0.90416667 -0.9 -0.89583333 -0.89166667 -0.8875 -0.88333333 -0.87916667 -0.875 -0.87083333 -0.86666667 -0.8625 -0.85833333 -0.85416667 -0.85 -0.84583333 -0.84166667 -0.8375 -0.83333333 -0.82916667 -0.825 -0.82083333 -0.81666667 -0.8125 -0.80833333 -0.80416667 -0.8 -0.79583333 -0.79166667 -0.7875 -0.78333333 -0.77916667 -0.775 -0.77083333 -0.76666667 -0.7625 -0.75833333 -0.75416667 -0.75 -0.74583333 -0.74166667 -0.7375 -0.73333333 -0.72916667 -0.725 -0.72083333 -0.71666667 -0.7125 -0.70833333 -0.70416667 -0.7 -0.69583333 -0.69166667 -0.6875 -0.68333333 -0.67916667 -0.675 -0.67083333 -0.66666667 -0.6625 -0.65833333 -0.65416667 -0.65 -0.64583333 -0.64166667 -0.6375 -0.63333333 -0.62916667 -0.625 -0.62083333 -0.61666667 -0.6125 -0.60833333 -0.60416667 -0.6 -0.59583333 -0.59166667 -0.5875 -0.58333333 -0.57916667 -0.575 -0.57083333 -0.56666667 -0.5625 -0.55833333 -0.55416667 -0.55 -0.54583333 -0.54166667 -0.5375 -0.53333333 -0.52916667 -0.525 -0.52083333 -0.51666667 -0.5125 -0.50833333 -0.50416667 -0.5 -0.49583333 -0.49166667 -0.4875 -0.48333333 -0.47916667 -0.475 -0.47083333 -0.46666667 -0.4625 -0.45833333 -0.45416667 -0.45 -0.44583333 -0.44166667 -0.4375 -0.43333333 -0.42916667 -0.425 -0.42083333 -0.41666667 -0.4125 -0.40833333 -0.40416667 -0.4 -0.39583333 -0.39166667 -0.3875 -0.38333333 -0.37916667 -0.375 -0.37083333 -0.36666667 -0.3625 -0.35833333 -0.35416667 -0.35 -0.34583333 -0.34166667 -0.3375 -0.33333333 -0.32916667 -0.325 -0.32083333 -0.31666667 -0.3125 -0.30833333 -0.30416667 -0.3 -0.29583333 -0.29166667 -0.2875 -0.28333333 -0.27916667 -0.275 -0.27083333 -0.26666667 -0.2625 -0.25833333 -0.25416667 -0.25 -0.24583333 -0.24166667 -0.2375 -0.23333333 -0.22916667 -0.225 -0.22083333 -0.21666667 -0.2125 -0.20833333 -0.20416667 -0.2 -0.19583333 -0.19166667 -0.1875 -0.18333333 -0.17916667 -0.175 -0.17083333 -0.16666667 -0.1625 -0.15833333 -0.15416667 -0.15 -0.14583333 -0.14166667 -0.1375 -0.13333333 -0.12916667 -0.125 -0.12083333 -0.11666667 -0.1125 -0.10833333 -0.10416667 -0.1 -0.09583333 -0.09166667 -0.0875 -0.08333333 -0.07916667 -0.075 -0.07083333 -0.06666667 -0.0625 -0.05833333 -0.05416667 -0.05 -0.04583333 -0.04166667 -0.0375 -0.03333333 -0.02916667 -0.025 -0.02083333 -0.01666667 -0.0125 -0.00833333 -0.00416667 0 0 0 0 0 0
  line L74 (18.6655, -5.1527) -> (18.6648, -5.1525)
  line L75 (18.6648, -5.1525) -> (18.074, -4.9894)
  arc A38 (18.074, -4.9894) -> (18.3692, -3.7599) centre (0, 0) ccw
  line L76 (18.3692, -3.7599) -> (18.9697, -3.8828)
  line L77 (18.9697, -3.8828) -> (18.9704, -3.8829)
  spline S38 degree 5 poles (18.9704, -3.8829) (18.9704, -3.8829) (18.9706, -3.883) (18.9708, -3.883) (18.9712, -3.8831) (18.9718, -3.8832) (18.9725, -3.8833) (18.9733, -3.8835) (18.9742, -3.8836) (18.9751, -3.8838) (18.9761, -3.884) (18.9773, -3.8842) (18.9785, -3.8844) (18.9798, -3.8846) (18.9811, -3.8848) (18.9826, -3.8851) (18.9841, -3.8853) (18.9858, -3.8856) (18.9875, -3.8859) (18.9892, -3.8862) (18.9911, -3.8865) (18.993, -3.8868) (18.9951, -3.8871) (18.9972, -3.8874) (18.9993, -3.8877) (19.0016, -3.888) (19.0039, -3.8884) (19.0063, -3.8887) (19.0088, -3.889) (19.0113, -3.8894) (19.0139, -3.8898) (19.0166, -3.8901) (19.0194, -3.8905) (19.0222, -3.8908) (19.0251, -3.8912) (19.0281, -3.8916) (19.0311, -3.892) (19.0342, -3.8923) (19.0374, -3.8927) (19.0406, -3.8931) (19.0439, -3.8935) (19.0473, -3.8939) (19.0507, -3.8942) (19.0542, -3.8946) (19.0578, -3.895) (19.0615, -3.8954) (19.0652, -3.8958) (19.0689, -3.8962) (19.0727, -3.8965) (19.0766, -3.8969) (19.0806, -3.8973) (19.0846, -3.8977) (19.0887, -3.898) (19.0928, -3.8984) (19.097, -3.8988) (19.1013, -3.8992) (19.1056, -3.8995) (19.11, -3.8999) (19.1144, -3.9002) (19.1189, -3.9006) (19.1235, -3.9009) (19.1281, -3.9013) (19.1327, -3.9016) (19.1375, -3.902) (19.1423, -3.9023) (19.1471, -3.9026) (19.152, -3.9029) (19.157, -3.9032) (19.162, -3.9035) (19.167, -3.9039) (19.1721, -3.9041) (19.1773, -3.9044) (19.1825, -3.9047) (19.1878, -3.905) (19.1932, -3.9053) (19.1985, -3.9055) (19.204, -3.9058) (19.2095, -3.906) (19.215, -3.9063) (19.2206, -3.9065) (19.2263, -3.9067) (19.232, -3.9069) (19.2377, -3.9071) (19.2435, -3.9073) (19.2494, -3.9075) (19.2553, -3.9077) (19.2612, -3.9079) (19.2672, -3.908) (19.2733, -3.9082) (19.2794, -3.9083) (19.2855, -3.9085) (19.2917, -3.9086) (19.2979, -3.9087) (19.3042, -3.9088) (19.3106, -3.9089) (19.317, -3.909) (19.3234, -3.9091) (19.3299, -3.9091) (19.3364, -3.9092) (19.343, -3.9092) (19.3496, -3.9093) (19.3563, -3.9093) (19.363, -3.9093) (19.3697, -3.9093) (19.3765, -3.9093) (19.3834, -3.9092) (19.3903, -3.9092) (19.3972, -3.9091) (19.4042, -3.9091) (19.4112, -3.909) (19.4183, -3.9089) (19.4254, -3.9088) (19.4325, -3.9087) (19.4397, -3.9085) (19.447, -3.9084) (19.4542, -3.9082) (19.4616, -3.9081) (19.4689, -3.9079) (19.4763, -3.9077) (19.4838, -3.9075) (19.4913, -3.9073) (19.4988, -3.907) (19.5064, -3.9068) (19.514, -3.9065) (19.5216, -3.9062) (19.5293, -3.9059) (19.5371, -3.9056) (19.5448, -3.9053) (19.5527, -3.905) (19.5605, -3.9046) (19.5684, -3.9043) (19.5763, -3.9039) (19.5843, -3.9035) (19.5923, -3.9031) (19.6004, -3.9027) (19.6085, -3.9022) (19.6166, -3.9018) (19.6248, -3.9013) (19.633, -3.9008) (19.6412, -3.9003) (19.6495, -3.8998) (19.6578, -3.8992) (19.6661, -3.8987) (19.6745, -3.8981) (19.683, -3.8975) (19.6914, -3.8969) (19.6999, -3.8963) (19.7084, -3.8957) (19.717, -3.8951) (19.7256, -3.8944) (19.7343, -3.8937) (19.7429, -3.893) (19.7517, -3.8923) (19.7604, -3.8916) (19.7692, -3.8908) (19.778, -3.89) (19.7869, -3.8893) (19.7958, -3.8885) (19.8047, -3.8876) (19.8136, -3.8868) (19.8226, -3.886) (19.8317, -3.8851) (19.8407, -3.8842) (19.8498, -3.8833) (19.8589, -3.8824) (19.8681, -3.8814) (19.8773, -3.8805) (19.8865, -3.8795) (19.8958, -3.8785) (19.9051, -3.8775) (19.9144, -3.8765) (19.9237, -3.8754) (19.9331, -3.8743) (19.9426, -3.8733) (19.952, -3.8722) (19.9615, -3.871) (19.971, -3.8699) (19.9806, -3.8687) (19.9901, -3.8675) (19.9997, -3.8663) (20.0094, -3.8651) (20.0191, -3.8639) (20.0288, -3.8626) (20.0385, -3.8614) (20.0483, -3.8601) (20.0581, -3.8588) (20.0679, -3.8574) (20.0777, -3.8561) (20.0876, -3.8547) (20.0975, -3.8533) (20.1075, -3.8519) (20.1175, -3.8505) (20.1275, -3.849) (20.1375, -3.8476) (20.1476, -3.8461) (20.1577, -3.8446) (20.1678, -3.843) (20.1779, -3.8415) (20.1881, -3.8399) (20.1983, -3.8383) (20.2085, -3.8367) (20.2188, -3.8351) (20.2291, -3.8334) (20.2394, -3.8318) (20.2498, -3.8301) (20.2601, -3.8284) (20.2705, -3.8267) (20.281, -3.8249) (20.2914, -3.8231) (20.3019, -3.8213) (20.3124, -3.8195) (20.323, -3.8177) (20.3335, -3.8158) (20.3441, -3.814) (20.3547, -3.8121) (20.3654, -3.8102) (20.3761, -3.8082) (20.3868, -3.8063) (20.3975, -3.8043) (20.4082, -3.8023) (20.419, -3.8003) (20.4298, -3.7982) (20.4406, -3.7962) (20.4515, -3.7941) (20.4624, -3.792) (20.4733, -3.7898) (20.4842, -3.7877) (20.4952, -3.7855) (20.5061, -3.7833) (20.5171, -3.7811) (20.5282, -3.7789) (20.5392, -3.7766) (20.5503, -3.7743) (20.5614, -3.772) (20.5725, -3.7697) (20.5837, -3.7674) (20.5948, -3.765) (20.606, -3.7626) (20.6173, -3.7602) (20.6285, -3.7578) (20.6398, -3.7553) (20.6488, -3.7533) (20.6556, -3.7519) (20.6601, -3.7508) (20.6624, -3.7503) knots 0 0 0 0 0 0 0.00416667 0.00833333 0.0125 0.01666667 0.02083333 0.025 0.02916667 0.03333333 0.0375 0.04166667 0.04583333 0.05 0.05416667 0.05833333 0.0625 0.06666667 0.07083333 0.075 0.07916667 0.08333333 0.0875 0.09166667 0.09583333 0.1 0.10416667 0.10833333 0.1125 0.11666667 0.12083333 0.125 0.12916667 0.13333333 0.1375 0.14166667 0.14583333 0.15 0.15416667 0.15833333 0.1625 0.16666667 0.17083333 0.175 0.17916667 0.18333333 0.1875 0.19166667 0.19583333 0.2 0.20416667 0.20833333 0.2125 0.21666667 0.22083333 0.225 0.22916667 0.23333333 0.2375 0.24166667 0.24583333 0.25 0.25416667 0.25833333 0.2625 0.26666667 0.27083333 0.275 0.27916667 0.28333333 0.2875 0.29166667 0.29583333 0.3 0.30416667 0.30833333 0.3125 0.31666667 0.32083333 0.325 0.32916667 0.33333333 0.3375 0.34166667 0.34583333 0.35 0.35416667 0.35833333 0.3625 0.36666667 0.37083333 0.375 0.37916667 0.38333333 0.3875 0.39166667 0.39583333 0.4 0.40416667 0.40833333 0.4125 0.41666667 0.42083333 0.425 0.42916667 0.43333333 0.4375 0.44166667 0.44583333 0.45 0.45416667 0.45833333 0.4625 0.46666667 0.47083333 0.475 0.47916667 0.48333333 0.4875 0.49166667 0.49583333 0.5 0.50416667 0.50833333 0.5125 0.51666667 0.52083333 0.525 0.52916667 0.53333333 0.5375 0.54166667 0.54583333 0.55 0.55416667 0.55833333 0.5625 0.56666667 0.57083333 0.575 0.57916667 0.58333333 0.5875 0.59166667 0.59583333 0.6 0.60416667 0.60833333 0.6125 0.61666667 0.62083333 0.625 0.62916667 0.63333333 0.6375 0.64166667 0.64583333 0.65 0.65416667 0.65833333 0.6625 0.66666667 0.67083333 0.675 0.67916667 0.68333333 0.6875 0.69166667 0.69583333 0.7 0.70416667 0.70833333 0.7125 0.71666667 0.72083333 0.725 0.72916667 0.73333333 0.7375 0.74166667 0.74583333 0.75 0.75416667 0.75833333 0.7625 0.76666667 0.77083333 0.775 0.77916667 0.78333333 0.7875 0.79166667 0.79583333 0.8 0.80416667 0.80833333 0.8125 0.81666667 0.82083333 0.825 0.82916667 0.83333333 0.8375 0.84166667 0.84583333 0.85 0.85416667 0.85833333 0.8625 0.86666667 0.87083333 0.875 0.87916667 0.88333333 0.8875 0.89166667 0.89583333 0.9 0.90416667 0.90833333 0.9125 0.91666667 0.92083333 0.925 0.92916667 0.93333333 0.9375 0.94166667 0.94583333 0.95 0.95416667 0.95833333 0.9625 0.96666667 0.97083333 0.975 0.97916667 0.98333333 0.9875 0.99166667 0.99583333 1 1 1 1 1 1
  arc A39 (20.6624, -3.7503) -> (20.81, -2.8182) centre (0, 0) ccw
  spline S39 degree 5 poles (20.81, -2.8182) (20.808, -2.8171) (20.804, -2.8147) (20.798, -2.8112) (20.7901, -2.8065) (20.7801, -2.8007) (20.7702, -2.7949) (20.7602, -2.7892) (20.7503, -2.7834) (20.7404, -2.7777) (20.7305, -2.772) (20.7207, -2.7664) (20.7108, -2.7608) (20.701, -2.7552) (20.6912, -2.7496) (20.6814, -2.7441) (20.6716, -2.7386) (20.6618, -2.7331) (20.6521, -2.7277) (20.6424, -2.7222) (20.6326, -2.7168) (20.6229, -2.7115) (20.6133, -2.7061) (20.6036, -2.7008) (20.594, -2.6956) (20.5843, -2.6903) (20.5747, -2.6851) (20.5652, -2.6799) (20.5556, -2.6747) (20.546, -2.6696) (20.5365, -2.6645) (20.527, -2.6594) (20.5175, -2.6543) (20.508, -2.6493) (20.4986, -2.6443) (20.4891, -2.6393) (20.4797, -2.6344) (20.4703, -2.6295) (20.4609, -2.6246) (20.4516, -2.6197) (20.4422, -2.6149) (20.4329, -2.6101) (20.4236, -2.6053) (20.4143, -2.6006) (20.4051, -2.5958) (20.3958, -2.5912) (20.3866, -2.5865) (20.3774, -2.5818) (20.3683, -2.5772) (20.3591, -2.5727) (20.35, -2.5681) (20.3409, -2.5636) (20.3318, -2.5591) (20.3227, -2.5546) (20.3137, -2.5502) (20.3046, -2.5458) (20.2956, -2.5414) (20.2867, -2.537) (20.2777, -2.5327) (20.2688, -2.5284) (20.2599, -2.5241) (20.251, -2.5199) (20.2421, -2.5156) (20.2333, -2.5114) (20.2245, -2.5073) (20.2157, -2.5031) (20.2069, -2.499) (20.1981, -2.495) (20.1894, -2.4909) (20.1807, -2.4869) (20.172, -2.4829) (20.1634, -2.4789) (20.1548, -2.475) (20.1462, -2.471) (20.1376, -2.4672) (20.1291, -2.4633) (20.1205, -2.4595) (20.112, -2.4557) (20.1036, -2.4519) (20.0951, -2.4481) (20.0867, -2.4444) (20.0783, -2.4407) (20.0699, -2.437) (20.0616, -2.4334) (20.0533, -2.4298) (20.045, -2.4262) (20.0367, -2.4226) (20.0285, -2.4191) (20.0203, -2.4156) (20.0121, -2.4121) (20.0039, -2.4086) (19.9958, -2.4052) (19.9877, -2.4018) (19.9797, -2.3984) (19.9716, -2.3951) (19.9636, -2.3918) (19.9556, -2.3885) (19.9477, -2.3852) (19.9398, -2.382) (19.9319, -2.3788) (19.924, -2.3756) (19.9162, -2.3724) (19.9084, -2.3693) (19.9006, -2.3662) (19.8929, -2.3631) (19.8851, -2.3601) (19.8775, -2.357) (19.8698, -2.354) (19.8622, -2.3511) (19.8546, -2.3481) (19.847, -2.3452) (19.8395, -2.3423) (19.832, -2.3394) (19.8246, -2.3366) (19.8171, -2.3338) (19.8098, -2.331) (19.8024, -2.3282) (19.7951, -2.3255) (19.7878, -2.3228) (19.7805, -2.3201) (19.7733, -2.3175) (19.7661, -2.3148) (19.7589, -2.3122) (19.7518, -2.3097) (19.7447, -2.3071) (19.7377, -2.3046) (19.7306, -2.3021) (19.7237, -2.2996) (19.7167, -2.2971) (19.7098, -2.2947) (19.7029, -2.2923) (19.6961, -2.29) (19.6893, -2.2876) (19.6825, -2.2853) (19.6758, -2.283) (19.6691, -2.2807) (19.6624, -2.2785) (19.6558, -2.2763) (19.6492, -2.2741) (19.6427, -2.2719) (19.6362, -2.2698) (19.6297, -2.2676) (19.6233, -2.2655) (19.6169, -2.2635) (19.6106, -2.2614) (19.6043, -2.2594) (19.598, -2.2574) (19.5918, -2.2555) (19.5856, -2.2535) (19.5795, -2.2516) (19.5734, -2.2497) (19.5673, -2.2478) (19.5613, -2.246) (19.5553, -2.2442) (19.5494, -2.2424) (19.5435, -2.2406) (19.5377, -2.2388) (19.5319, -2.2371) (19.5261, -2.2354) (19.5204, -2.2337) (19.5147, -2.2321) (19.5091, -2.2305) (19.5035, -2.2289) (19.498, -2.2273) (19.4925, -2.2257) (19.4871, -2.2242) (19.4817, -2.2227) (19.4763, -2.2212) (19.471, -2.2197) (19.4658, -2.2183) (19.4606, -2.2169) (19.4554, -2.2155) (19.4503, -2.2141) (19.4452, -2.2128) (19.4402, -2.2115) (19.4353, -2.2102) (19.4304, -2.2089) (19.4255, -2.2076) (19.4207, -2.2064) (19.4159, -2.2052) (19.4112, -2.204) (19.4066, -2.2028) (19.402, -2.2017) (19.3974, -2.2006) (19.393, -2.1995) (19.3885, -2.1984) (19.3841, -2.1973) (19.3798, -2.1963) (19.3755, -2.1953) (19.3713, -2.1943) (19.3671, -2.1933) (19.363, -2.1924) (19.359, -2.1915) (19.355, -2.1906) (19.3511, -2.1897) (19.3472, -2.1888) (19.3434, -2.188) (19.3396, -2.1872) (19.3359, -2.1864) (19.3323, -2.1856) (19.3287, -2.1848) (19.3252, -2.1841) (19.3217, -2.1834) (19.3183, -2.1827) (19.315, -2.182) (19.3117, -2.1813) (19.3085, -2.1807) (19.3054, -2.1801) (19.3023, -2.1795) (19.2993, -2.1789) (19.2964, -2.1783) (19.2935, -2.1778) (19.2907, -2.1772) (19.288, -2.1767) (19.2853, -2.1762) (19.2827, -2.1758) (19.2802, -2.1753) (19.2777, -2.1749) (19.2753, -2.1745) (19.273, -2.1741) (19.2708, -2.1737) (19.2686, -2.1733) (19.2665, -2.173) (19.2645, -2.1726) (19.2626, -2.1723) (19.2607, -2.172) (19.259, -2.1718) (19.2573, -2.1715) (19.2556, -2.1712) (19.2541, -2.171) (19.2526, -2.1708) (19.2512, -2.1706) (19.2499, -2.1704) (19.2487, -2.1702) (19.2476, -2.1701) (19.2466, -2.1699) (19.2456, -2.1698) (19.2447, -2.1697) (19.244, -2.1696) (19.2433, -2.1695) (19.2427, -2.1694) (19.2423, -2.1694) (19.242, -2.1693) (19.2418, -2.1693) (19.2418, -2.1693) knots -1 -1 -1 -1 -1 -1 -0.99583333 -0.99166667 -0.9875 -0.98333333 -0.97916667 -0.975 -0.97083333 -0.96666667 -0.9625 -0.95833333 -0.95416667 -0.95 -0.94583333 -0.94166667 -0.9375 -0.93333333 -0.92916667 -0.925 -0.92083333 -0.91666667 -0.9125 -0.90833333 -0.90416667 -0.9 -0.89583333 -0.89166667 -0.8875 -0.88333333 -0.87916667 -0.875 -0.87083333 -0.86666667 -0.8625 -0.85833333 -0.85416667 -0.85 -0.84583333 -0.84166667 -0.8375 -0.83333333 -0.82916667 -0.825 -0.82083333 -0.81666667 -0.8125 -0.80833333 -0.80416667 -0.8 -0.79583333 -0.79166667 -0.7875 -0.78333333 -0.77916667 -0.775 -0.77083333 -0.76666667 -0.7625 -0.75833333 -0.75416667 -0.75 -0.74583333 -0.74166667 -0.7375 -0.73333333 -0.72916667 -0.725 -0.72083333 -0.71666667 -0.7125 -0.70833333 -0.70416667 -0.7 -0.69583333 -0.69166667 -0.6875 -0.68333333 -0.67916667 -0.675 -0.67083333 -0.66666667 -0.6625 -0.65833333 -0.65416667 -0.65 -0.64583333 -0.64166667 -0.6375 -0.63333333 -0.62916667 -0.625 -0.62083333 -0.61666667 -0.6125 -0.60833333 -0.60416667 -0.6 -0.59583333 -0.59166667 -0.5875 -0.58333333 -0.57916667 -0.575 -0.57083333 -0.56666667 -0.5625 -0.55833333 -0.55416667 -0.55 -0.54583333 -0.54166667 -0.5375 -0.53333333 -0.52916667 -0.525 -0.52083333 -0.51666667 -0.5125 -0.50833333 -0.50416667 -0.5 -0.49583333 -0.49166667 -0.4875 -0.48333333 -0.47916667 -0.475 -0.47083333 -0.46666667 -0.4625 -0.45833333 -0.45416667 -0.45 -0.44583333 -0.44166667 -0.4375 -0.43333333 -0.42916667 -0.425 -0.42083333 -0.41666667 -0.4125 -0.40833333 -0.40416667 -0.4 -0.39583333 -0.39166667 -0.3875 -0.38333333 -0.37916667 -0.375 -0.37083333 -0.36666667 -0.3625 -0.35833333 -0.35416667 -0.35 -0.34583333 -0.34166667 -0.3375 -0.33333333 -0.32916667 -0.325 -0.32083333 -0.31666667 -0.3125 -0.30833333 -0.30416667 -0.3 -0.29583333 -0.29166667 -0.2875 -0.28333333 -0.27916667 -0.275 -0.27083333 -0.26666667 -0.2625 -0.25833333 -0.25416667 -0.25 -0.24583333 -0.24166667 -0.2375 -0.23333333 -0.22916667 -0.225 -0.22083333 -0.21666667 -0.2125 -0.20833333 -0.20416667 -0.2 -0.19583333 -0.19166667 -0.1875 -0.18333333 -0.17916667 -0.175 -0.17083333 -0.16666667 -0.1625 -0.15833333 -0.15416667 -0.15 -0.14583333 -0.14166667 -0.1375 -0.13333333 -0.12916667 -0.125 -0.12083333 -0.11666667 -0.1125 -0.10833333 -0.10416667 -0.1 -0.09583333 -0.09166667 -0.0875 -0.08333333 -0.07916667 -0.075 -0.07083333 -0.06666667 -0.0625 -0.05833333 -0.05416667 -0.05 -0.04583333 -0.04166667 -0.0375 -0.03333333 -0.02916667 -0.025 -0.02083333 -0.01666667 -0.0125 -0.00833333 -0.00416667 0 0 0 0 0 0
  line L78 (19.2418, -2.1693) -> (19.2411, -2.1692)
  line L79 (19.2411, -2.1692) -> (18.632, -2.1005)
  arc A40 (18.632, -2.1005) -> (18.7312, -0.84) centre (0, 0) ccw
  line L80 (18.7312, -0.84) -> (19.3435, -0.8675)
  line L81 (19.3435, -0.8675) -> (19.3442, -0.8675)